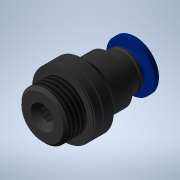
# Autodesk Inventor part: 186106 QS-G1/8-4-I
Saved by Autodesk Inventor 2021 (Build 250183000, 183)
## iProperties
Created: 2026-09-15
Part Number: 186106 QS-G1/8-4-I
Material: Generic
Catalog Web Link: www.3dfindit.com
Description: QS-G-I-push-in fitting
Vendor: FESTO
Document SubType Name: Modeling
Designer: psAdmin
Manufacturer: FESTO
Mass: 7.7 g
Surface Area: 11.4725 cm^2
Volume: 1.33545 cm^3
Density: 1 g/cm^3
Appearance: PSOLRGB-176-176-176
Category: PARTsolutions
Company: FESTO
Title: 186106 QS-G1/8-4-I
Author: Cadenas PARTsolutions
Comments: push-in fitting
PSOL_IDENT_0: {$CADENAS_DATA/23d-libs/festo/parts/q/qs/qs_g_i.prj},176 {VTYP=3D},{NB=186106 QS-G1/8-4-I},{LINA=186
PSOL_IDENT_1: 106 QS-G1/8-4-I},{NN=QS-G-I},{DATE=10.08.2026 11:26:37},{GEOMDATE=22.05.2025 14:11:35},{VERSION=},{L
PSOL_IDENT_2: INEID=10},{WBVAR=},{WBNUMERIC=}  {NB=186106 QS-G1/8-4-I},{LINA=186106 QS-G1/8-4-I},{KT=DUMMY},{TNR=1
PSOL_IDENT_3: 86106},{TYP=QS-G1/8-4-I},{D1=G1/8},{NENN=2.600},{D2=4.000},{D5=13.000},{L1=19.500},{L2=4.200},{SW=2.
PSOL_IDENT_4: 500},{T=14.900},{CNSMASSEXACT=0.00770},{D1N=9.728},{Z=9.900},{K1=13.000},{GB=1.900},{D6=9.700},{D7=7
PSOL_IDENT_5: .500},{L7=3.100},{GTIN=4052568039196},{ZOLL=1/8},{FDTQS=-},{FDTQSCMSH=-},{REACH=Ja},{REACHSVHC=Ja},{
PSOL_IDENT_6: REACHHAZSUBS=7439-92-1},{REACHSCIP=3732228b-b396-49b9-8f0d-ee75d35d3f40},{REACHVALDATE=05.03.2025}
NB: 186106 QS-G1/8-4-I
NN: QS-G-I
NT: push-in fitting
NBSYN: $TNR. $TYP.
LINA: 186106 QS-G1/8-4-I
CATALOG: Festo
TNR: 186106
TYP: QS-G1/8-4-I
D1: G1/8
NENN: 2.6
D2: 4
D5: 13
L1: 19.5
L2: 4.2
SW: 2.5
T: 14.9
CNSMASSEXACT: 0.0077
GTIN: 4052568039196
REACH: Yes
REACHSVHC: Yes
REACHHAZSUBS: 7439-92-1
REACHVALDATE: 05.03.2025
SUPPLIER: FESTO
ARTICLENO: 186106 QS-G1/8-4-I
BOMINFO: 186106 QS-G1/8-4-I
CREATOR: CADENAS GmbH
Autodesk Inventor part; units mm, degrees
sketch "Sketch_4" plane through (0, 0, 0) normal (1, 0, 0) x (0, 1, 0)
  line L0 (0, -15.3) -> (0, -1.9)
  line L1 (0, -1.9) -> (4.85, -1.9)
  line L2 (4.85, -1.9) -> (4.85, -9.3959)
  line L3 (4.85, -9.3959) -> (4.15, -9.8)
  line L4 (4.15, -9.8) -> (3.75, -9.8)
  line L5 (3.75, -9.8) -> (3.75, -11.95)
  line L6 (3.75, -11.95) -> (3.55, -12.15)
  line L7 (3.55, -12.15) -> (3.75, -12.35)
  line L8 (3.75, -12.35) -> (3.75, -12.7586)
  line L9 (3.75, -12.7586) -> (3.6086, -12.9)
  line L10 (3.6086, -12.9) -> (2.7, -12.9)
  line L11 (2.7, -12.9) -> (2.7, -13.425)
  arc A0 (2.7, -13.425) -> (3.075, -13.8) centre (3.075, -13.425) ccw
  line L12 (3.075, -13.8) -> (4.95, -13.8)
  line L13 (4.95, -13.8) -> (4.95, -14.6649)
  arc A1 (4.7847, -14.8619) -> (4.95, -14.6649) centre (4.75, -14.6649) ccw
  line L14 (4.7847, -14.8619) -> (2.3, -15.3)
  line L15 (2.3, -15.3) -> (0, -15.3)
  line L16 (0, -15.3) -> (0, -1.9)
  constraints: 34 end point, 4 point on circle, 2 centre point
revolve "Revolution1" add sketch "Sketch_4" angle 360 about axis through (0, 0, -15.3) along (0, 0, -1)
sketch "Sketch_1" plane through (0, 0, 0) normal (1, 0, 0) x (0, 1, 0)
  line L0 (0, -10.4) -> (0, -1.9)
  line L1 (0, -1.9) -> (6.5, -1.9)
  line L2 (6.5, -1.9) -> (6.5, -3.9)
  line L3 (6.5, -3.9) -> (0, -10.4)
  line L4 (0, -10.4) -> (0, -1.9)
  constraints: 10 end point
revolve "Revolution2" add sketch "Sketch_1" angle 360 about axis through (0, 0, -10.4) along (0, 0, -1)
sketch "Sketch_5" plane through (0, 0, 0) normal (1, 0, 0) x (0, 1, 0)
  line L0 (0, -1.9) -> (0, 4.2)
  line L1 (0, 4.2) -> (4.283, 4.2)
  line L2 (4.283, 4.2) -> (4.864, 3.619)
  line L3 (4.864, 3.619) -> (4.864, 0)
  line L4 (4.864, 0) -> (6.2, 0)
  line L5 (6.2, 0) -> (6.2, -0.2)
  line L6 (6.2, -0.2) -> (6.5, -0.2)
  line L7 (6.5, -0.2) -> (6.5, -1.7)
  line L8 (6.5, -1.7) -> (6.2, -1.7)
  line L9 (6.2, -1.7) -> (6.2, -1.9)
  line L10 (6.2, -1.9) -> (0, -1.9)
  line L11 (0, -1.9) -> (0, 4.2)
  constraints: 24 end point
revolve "Revolution3" add sketch "Sketch_5" angle 360 about axis through (0, 0, -1.9) along (0, 0, -1)
thread "Thread1" size "G9.728x0.907" designation "G 1/8" class "A" standard "ISO Pipe Threads" full length
sketch "Sketch_6" plane through (0, 0, 0) normal (1, 0, 0) x (0, 1, 0)
  line L0 (0, -15.3) -> (0, 4.2)
  line L1 (0, 4.2) -> (2.4, 4.2)
  line L2 (2.4, 4.2) -> (1.3, 3.1)
  line L3 (1.3, 3.1) -> (1.3, -0.4)
  line L4 (1.3, -0.4) -> (2, -0.4)
  line L5 (2, -0.4) -> (2, -15)
  arc A0 (2, -15) -> (2.3, -15.3) centre (2.3, -15) ccw
  line L6 (2.3, -15.3) -> (0, -15.3)
  line L7 (0, -15.3) -> (0, 4.2)
  constraints: 16 end point, 2 point on circle, 1 centre point
revolve "Revolution4" cut sketch "Sketch_6" angle 360 about axis through (0, 0, -15.3) along (0, 0, -1)
sketch "Sketch_7" plane through (0, 0, 4.2) normal (0, 0, 1) x (1, 0, 0)
  line L0 (-1.25, -0.7217) -> (0, -1.4434)
  line L1 (0, -1.4434) -> (1.25, -0.7217)
  line L2 (1.25, -0.7217) -> (1.25, 0.7217)
  line L3 (1.25, 0.7217) -> (0, 1.4434)
  line L4 (0, 1.4434) -> (-1.25, 0.7217)
  line L5 (-1.25, 0.7217) -> (-1.25, -0.7217)
  constraints: 12 end point
extrude "Extrusion1" cut sketch "Sketch_7" against normal blind 4.6
ref_plane "ANBAU_XY" through (0, 0, 0) normal (0, 0, -1) x (1, 0, 0)
ref_plane "ANBAU_YZ" through (0, 0, 0) normal (1, 0, 0) x (0, -1, 0)
ref_plane "ANBAU_ZX" through (0, 0, 0) normal (0, -1, 0) x (0, 0, -1)
ref_plane "ANBAU_STD_XY" through (0, 0, 0) normal (0, 0, -1) x (1, 0, 0)
ref_plane "ANBAU_STD_YZ" through (0, 0, 0) normal (1, 0, 0) x (0, -1, 0)
ref_plane "ANBAU_STD_ZX" through (0, 0, 0) normal (0, -1, 0) x (0, 0, -1)
ref_plane "CP_XY" through (0, 0, -15.3) normal (0, 0, -1) x (1, 0, 0)
ref_plane "CP_YZ" through (0, 0, -15.3) normal (1, 0, 0) x (0, -1, 0)
ref_plane "CP_ZX" through (0, 0, -15.3) normal (0, -1, 0) x (0, 0, -1)
ref_plane "CPV_XY" through (0, 0, 0) normal (0, 0, -1) x (1, 0, 0)
ref_plane "CPV_YZ" through (0, 0, 0) normal (1, 0, 0) x (0, -1, 0)
ref_plane "CPV_ZX" through (0, 0, 0) normal (0, -1, 0) x (0, 0, -1)
ref_plane "CPV_ANBAU_XY" through (0, 0, 0) normal (0, 0, -1) x (1, 0, 0)
ref_plane "CPV_ANBAU_YZ" through (0, 0, 0) normal (1, 0, 0) x (0, -1, 0)
ref_plane "CPV_ANBAU_ZX" through (0, 0, 0) normal (0, -1, 0) x (0, 0, -1)
ref_plane "FDT_SCHLAUCH_XY" through (0, 0, -0.4) normal (0, 0, -1) x (1, 0, 0)
ref_plane "FDT_SCHLAUCH_YZ" through (0, 0, -0.4) normal (1, 0, 0) x (0, -1, 0)
ref_plane "FDT_SCHLAUCH_ZX" through (0, 0, -0.4) normal (0, -1, 0) x (0, 0, -1)
body "Solid1"
